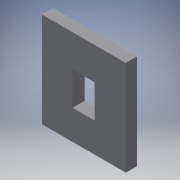
# Autodesk Inventor part: TapaFrontal
Saved by Autodesk Inventor 2017 (Build 210142000, 142)
## iProperties
Created: 2021-02-12
Part Number: TapaFrontal
Material: Generic
Document SubType Name: Modeling
Designer: USUARIO
Density: 1 g/cm^3
Appearance: Default
Author: USUARIO
Autodesk Inventor part; units mm, degrees
ref_plane "YZ Plane" through (0, 0, 0) normal (1, 0, 0) x (0, 1, 0)
ref_plane "XZ Plane" through (0, 0, 0) normal (0, 1, 0) x (-1, 0, 0)
ref_plane "XY Plane" through (0, 0, 0) normal (0, 0, 1) x (1, 0, 0)
sketch "Sketch1" plane through (0, 0, 0) normal (0, 1, 0) x (-1, 0, 0)
  line L0 (0, 0) -> (380, 0)
  line L1 (380, 0) -> (380, -430)
  line L2 (380, -430) -> (0, -430)
  line L3 (0, -430) -> (0, 0)
  line L4 (249.75, -140) -> (149.75, -140)
  line L5 (149.75, -140) -> (149.75, -290)
  line L6 (149.75, -290) -> (249.75, -290)
  line L7 (249.75, -290) -> (249.75, -140)
  dimension "d0" = 380
  dimension "d1" = 430
  dimension "d2" = 100
  dimension "d3" = 150
  dimension "d4" = 140
  dimension "d5" = 149.75
  constraints: 16 end point, 4 parallel, 2 horizontal, 2 perpendicular
  measures "d0" distance of L1.end L2.end
  measures "d1" distance of L0.end L1.end
  measures "d2" distance of L6.end L5.end
  measures "d3" distance of L5.end L4.end
  measures "d4" distance between parallel lines of L2 L6
  measures "d5" distance between parallel lines of L3 L5
extrude "Extrusion1" add sketch "Sketch1" along normal blind 50.8
sketch "Sketch5" plane through (0, 50.8, 0) normal (0, 1, 0) x (1, 0, 0)
  line L0 (-349.5, 38) -> (-50, 38)
  line L1 (-50, 38) -> (-50, 392)
  line L2 (-50, 392) -> (-349.5, 392)
  line L3 (-349.5, 392) -> (-349.5, 38)
  line L4 (-380, 0) -> (0, 0) projected
  line L5 (-380, 430) -> (-380, 0) projected
  line L6 (-249.75, 140) -> (-149.75, 140) projected
  line L7 (-149.75, 290) -> (-249.75, 290) projected
  line L8 (-249.75, 140) -> (-149.75, 140)
  line L9 (-149.75, 140) -> (-149.75, 290)
  line L10 (-149.75, 290) -> (-249.75, 290)
  line L11 (-249.75, 290) -> (-249.75, 140)
  dimension "d14" = 299.5
  dimension "d15" = 354
  dimension "d16" = 38
  dimension "d17" = 30.5
  constraints: 16 end point, 4 parallel, 2 horizontal, 2 perpendicular
  measures "d14" distance of L2.end L1.end
  measures "d15" distance of L1.end L0.end
  measures "d16" distance between parallel lines of L0 L4
  measures "d17" distance between parallel lines of L5 L3
extrude "Extrusion2" add sketch "Sketch5" along normal blind 5
body "Solid1"
